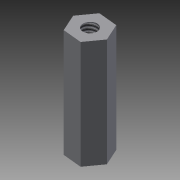
# Autodesk Inventor part: standoff
Saved by Autodesk Inventor 2015 (Build 190159000, 159)
## iProperties
Created: 2015-05-13
Part Number: standoff
Material: Generic
Document SubType Name: Modeling
Designer: Angelina
Density: 1 g/cm^3
Appearance: Default
Author: Angelina
Autodesk Inventor part; units mm, degrees
ref_plane "YZ Plane" through (0, 0, 0) normal (1, 0, 0) x (0, 1, 0)
ref_plane "XZ Plane" through (0, 0, 0) normal (0, 1, 0) x (-1, 0, 0)
ref_plane "XY Plane" through (0, 0, 0) normal (0, 0, 1) x (1, 0, 0)
sketch "Sketch1" plane through (0, 0, 0) normal (0, 1, 0) x (-1, 0, 0)
  line L0 (1.9345, 2.6954) -> (3.3015, -0.3277)
  line L1 (3.3015, -0.3277) -> (1.367, -3.0231)
  line L2 (1.367, -3.0231) -> (-1.9345, -2.6954)
  line L3 (-1.9345, -2.6954) -> (-3.3015, 0.3277)
  line L4 (-3.3015, 0.3277) -> (-1.367, 3.0231)
  line L5 (-1.367, 3.0231) -> (1.9345, 2.6954)
  point P0 (0, 0)
  point P1 (0, 0)
  constraints: 12 end point, 1 coincident, 13 other
extrude "Extrusion1" add sketch "Sketch1" along normal blind 19.05
sketch "Sketch2" plane through (0, 19.05, 0) normal (0, 1, 0) x (1, 0, 0)
  point P0 (0, 0)
  point P1 (0, 0)
  constraints: 1 coincident
hole "Hole1" at (0, 19.05, 0) direction (0, -1, 0) diameter 2.4892 end through all
body "Solid1"
